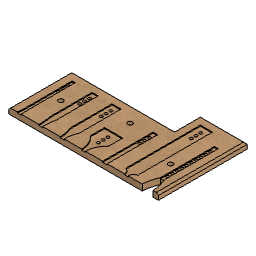
model (Autodesk Fusion 360 design; units mm, degrees)
Autodesk Fusion 360 part; units mm, degrees
(part 1 of 4)
sketch "scan" plane through (0, 0, 0) normal (0, 0, 1) x (1, 0, 0)
  spline S0 degree 3 poles (16.3721, 38.0071) (16.4657, 38.4045) (16.5594, 38.8018) (16.653, 39.1992) knots 0 0 0 0 1 1 1 1
  spline S1 degree 3 poles (24.0485, 109.3811) (21.8648, 109.3248) (19.6635, 109.4946) (17.4974, 109.2121) knots 0 0 0 0 1 1 1 1
  spline S2 degree 3 poles (17.4974, 109.2121) (17.1008, 109.1604) (16.6596, 108.8066) (16.6045, 108.4104) knots 0 0 0 0 1 1 1 1
  spline S3 degree 3 poles (16.6045, 108.4104) (16.3062, 106.2687) (16.4944, 104.0868) (16.4827, 101.9245) knots 0 0 0 0 1 1 1 1
  spline S4 degree 3 poles (16.4827, 101.9245) (16.4424, 94.5014) (16.447, 87.0781) (16.4485, 79.6549) knots 0 0 0 0 1 1 1 1
  spline S5 degree 3 poles (16.4485, 79.6549) (16.4488, 78.5036) (16.4235, 77.3507) (16.4881, 76.2012) knots 0 0 0 0 1 1 1 1
  spline S6 degree 3 poles (16.4881, 76.2012) (16.5002, 75.9869) (16.653, 75.7989) (16.6771, 75.5856) knots 0 0 0 0 1 1 1 1
  spline S7 degree 3 poles (16.6771, 75.5856) (16.7158, 75.2443) (16.6755, 74.8985) (16.6746, 74.555) knots 0 0 0 0 1 1 1 1
  spline S8 degree 3 poles (17.0021, 108.8537) (16.9862, 98.3384) (16.9774, 87.823) (16.9544, 77.3076) knots 0 0 0 0 1 1 1 1
  spline S9 degree 3 poles (16.9544, 77.3076) (16.9536, 76.9758) (16.9724, 76.6416) (16.9307, 76.3123) knots 0 0 0 0 1 1 1 1
  spline S10 degree 3 poles (16.9307, 76.3123) (16.8044, 75.3143) (16.5462, 74.3342) (16.4514, 73.3326) knots 0 0 0 0 1 1 1 1
  spline S11 degree 3 poles (16.4514, 73.3326) (16.3616, 72.3843) (16.3872, 71.4283) (16.378, 70.4757) knots 0 0 0 0 1 1 1 1
  spline S12 degree 3 poles (16.378, 70.4757) (16.3753, 70.1956) (16.3712, 69.9127) (16.4159, 69.6362) knots 0 0 0 0 1 1 1 1
  spline S13 degree 3 poles (16.4159, 69.6362) (16.5418, 68.859) (16.77, 68.1003) (16.8886, 67.322) knots 0 0 0 0 1 1 1 1
  spline S14 degree 3 poles (16.8886, 67.322) (16.9349, 67.018) (16.9083, 66.7072) (16.9093, 66.3996) knots 0 0 0 0 1 1 1 1
  spline S15 degree 3 poles (16.9093, 66.3996) (16.9325, 58.9199) (17.042, 51.4397) (16.9613, 43.9603) knots 0 0 0 0 1 1 1 1
  spline S16 degree 3 poles (16.9613, 43.9603) (16.9556, 43.4252) (16.6548, 42.9203) (16.6502, 42.3851) knots 0 0 0 0 1 1 1 1
  spline S17 degree 3 poles (16.6502, 42.3851) (16.6468, 41.9959) (16.8806, 41.6384) (16.938, 41.2534) knots 0 0 0 0 1 1 1 1
  spline S18 degree 3 poles (16.938, 41.2534) (16.9834, 40.9489) (16.9566, 40.6379) (16.9564, 40.3301) knots 0 0 0 0 1 1 1 1
  spline S19 degree 3 poles (16.9564, 40.3301) (16.9563, 40.2112) (16.9677, 40.0888) (16.9369, 39.9739) knots 0 0 0 0 1 1 1 1
  spline S20 degree 3 poles (16.9369, 39.9739) (16.8656, 39.7083) (16.7476, 39.4575) (16.653, 39.1992) knots 0 0 0 0 1 1 1 1
  spline S21 degree 3 poles (16.674, 74.3159) (16.7683, 73.9813) (16.9278, 73.6585) (16.9568, 73.3121) knots 0 0 0 0 1 1 1 1
  spline S22 degree 3 poles (16.9568, 73.3121) (17.0258, 72.4891) (16.9752, 71.6602) (16.9658, 70.8343) knots 0 0 0 0 1 1 1 1
  spline S23 degree 3 poles (16.9658, 70.8343) (16.9603, 70.3518) (16.993, 69.8634) (16.9124, 69.3876) knots 0 0 0 0 1 1 1 1
  spline S24 degree 3 poles (16.9124, 69.3876) (16.7951, 68.6953) (16.5155, 68.0387) (16.3757, 67.3506) knots 0 0 0 0 1 1 1 1
  spline S25 degree 3 poles (16.3757, 67.3506) (16.3264, 67.1081) (16.3472, 66.8563) (16.3477, 66.6089) knots 0 0 0 0 1 1 1 1
  spline S26 degree 3 poles (16.3477, 66.6089) (16.3626, 59.0903) (16.3279, 51.5712) (16.4218, 44.0531) knots 0 0 0 0 1 1 1 1
  spline S27 degree 3 poles (16.4218, 44.0531) (16.4288, 43.492) (16.6492, 42.9463) (16.6502, 42.3851) knots 0 0 0 0 1 1 1 1
  spline S28 degree 3 poles (16.6502, 42.3851) (16.6512, 41.79) (16.4763, 41.2067) (16.4279, 40.6135) knots 0 0 0 0 1 1 1 1
  spline S29 degree 3 poles (16.4279, 40.6135) (16.41, 40.3942) (16.4182, 40.1712) (16.4517, 39.9536) knots 0 0 0 0 1 1 1 1
  spline S30 degree 3 poles (16.4517, 39.9536) (16.5857, 39.0828) (16.8758, 38.2335) (16.9295, 37.3541) knots 0 0 0 0 1 1 1 1
  spline S31 degree 3 poles (16.9295, 37.3541) (17.0419, 35.5128) (16.9584, 33.6646) (16.9484, 31.8199) knots 0 0 0 0 1 1 1 1
  spline S32 degree 3 poles (16.9484, 31.8199) (16.9468, 31.5315) (16.9648, 31.2361) (16.8948, 30.9563) knots 0 0 0 0 1 1 1 1
  spline S33 degree 3 poles (16.8948, 30.9563) (16.8, 30.5773) (16.605, 30.2306) (16.4602, 29.8678) knots 0 0 0 0 1 1 1 1
  spline S34 degree 3 poles (16.3721, 38.0071) (16.4021, 37.3563) (16.4583, 36.7062) (16.4621, 36.0548) knots 0 0 0 0 1 1 1 1
  spline S35 degree 3 poles (16.4621, 36.0548) (16.4803, 32.9771) (16.3867, 29.8988) (16.4382, 26.8215) knots 0 0 0 0 1 1 1 1
  spline S36 degree 3 poles (16.4382, 26.8215) (16.4474, 26.27) (16.5754, 25.7268) (16.644, 25.1795) knots 0 0 0 0 1 1 1 1
  spline S37 degree 3 poles (16.4626, 31.0645) (16.6175, 30.6597) (16.8137, 30.2684) (16.9274, 29.8501) knots 0 0 0 0 1 1 1 1
  spline S38 degree 3 poles (16.9274, 29.8501) (16.977, 29.6674) (16.9469, 29.4717) (16.9467, 29.2823) knots 0 0 0 0 1 1 1 1
  spline S39 degree 3 poles (16.9467, 29.2823) (16.9452, 28.2612) (16.9973, 27.2375) (16.9222, 26.2193) knots 0 0 0 0 1 1 1 1
  spline S40 degree 3 poles (16.9222, 26.2193) (16.8958, 25.8615) (16.683, 25.5362) (16.644, 25.1795) knots 0 0 0 0 1 1 1 1
  spline S41 degree 3 poles (16.644, 25.1795) (16.5882, 24.6699) (16.6796, 24.1528) (16.64, 23.6417) knots 0 0 0 0 1 1 1 1
  spline S42 degree 3 poles (16.64, 23.6417) (16.6178, 23.3553) (16.4873, 23.0849) (16.4597, 22.799) knots 0 0 0 0 1 1 1 1
  spline S43 degree 3 poles (16.4597, 22.799) (16.3985, 22.1675) (16.3449, 21.5313) (16.3743, 20.8976) knots 0 0 0 0 1 1 1 1
  spline S44 degree 3 poles (16.3743, 20.8976) (16.3993, 20.358) (16.5395, 19.83) (16.6221, 19.2962) knots 0 0 0 0 1 1 1 1
  spline S45 degree 3 poles (15.8229, 0.017) (15.863, 0.507) (15.9277, 0.9956) (15.9433, 1.487) knots 0 0 0 0 1 1 1 1
  spline S46 degree 3 poles (15.9433, 1.487) (16.1106, 6.7611) (16.1154, 12.0409) (16.3715, 17.3114) knots 0 0 0 0 1 1 1 1
  spline S47 degree 3 poles (16.3715, 17.3114) (16.4372, 18.6632) (16.7727, 19.9893) (16.9077, 21.336) knots 0 0 0 0 1 1 1 1
  spline S48 degree 3 poles (16.9077, 21.336) (16.9543, 21.8005) (16.9692, 22.2727) (16.9154, 22.7365) knots 0 0 0 0 1 1 1 1
  spline S49 degree 3 poles (16.9154, 22.7365) (16.879, 23.0498) (16.7318, 23.3399) (16.64, 23.6417) knots 0 0 0 0 1 1 1 1
  spline S50 degree 3 poles (16.33, 0.0256) (16.4989, 5.1912) (16.6867, 10.3561) (16.8367, 15.5223) knots 0 0 0 0 1 1 1 1
  spline S51 degree 3 poles (16.8367, 15.5223) (16.8574, 16.2368) (16.8899, 16.9534) (16.842, 17.6666) knots 0 0 0 0 1 1 1 1
  spline S52 degree 3 poles (16.842, 17.6666) (16.8169, 18.041) (16.6931, 18.4021) (16.6187, 18.7699) knots 0 0 0 0 1 1 1 1
  spline S53 degree 3 poles (23.6843, 24.1713) (23.7833, 24.7166) (23.8823, 25.2618) (23.9813, 25.8071) knots 0 0 0 0 1 1 1 1
  spline S54 degree 3 poles (23.946, 50.5495) (23.8732, 50.1915) (23.7551, 49.8398) (23.7276, 49.4756) knots 0 0 0 0 1 1 1 1
  spline S55 degree 3 poles (23.7276, 49.4756) (23.6586, 48.5602) (23.6607, 47.6406) (23.6575, 46.7227) knots 0 0 0 0 1 1 1 1
  spline S56 degree 3 poles (23.6575, 46.7227) (23.6433, 42.5512) (23.6628, 38.3797) (23.6757, 34.2082) knots 0 0 0 0 1 1 1 1
  spline S57 degree 3 poles (23.6757, 34.2082) (23.6765, 33.9424) (23.637, 33.6698) (23.6985, 33.4112) knots 0 0 0 0 1 1 1 1
  spline S58 degree 3 poles (23.6985, 33.4112) (23.8246, 32.8813) (24.0546, 32.3816) (24.2327, 31.8669) knots 0 0 0 0 1 1 1 1
  spline S59 degree 3 poles (24.1935, 40.1987) (24.0636, 40.2075) (23.9098, 40.1496) (23.8037, 40.2251) knots 0 0 0 0 1 1 1 1
  spline S60 degree 3 poles (23.8037, 40.2251) (23.7167, 40.287) (23.7491, 40.4314) (23.7218, 40.5345) knots 0 0 0 0 1 1 1 1
  spline S61 degree 3 poles (24.2007, 33.6134) (24.0442, 33.0019) (23.8612, 32.3965) (23.7312, 31.7788) knots 0 0 0 0 1 1 1 1
  spline S62 degree 3 poles (23.7312, 31.7788) (23.6859, 31.5639) (23.6512, 31.3404) (23.6764, 31.1222) knots 0 0 0 0 1 1 1 1
  spline S63 degree 3 poles (23.6764, 31.1222) (23.7323, 30.6384) (23.9641, 30.1784) (23.9723, 29.6914) knots 0 0 0 0 1 1 1 1
  spline S64 degree 3 poles (23.9723, 29.6914) (23.9792, 29.2772) (23.7818, 28.8841) (23.7207, 28.4744) knots 0 0 0 0 1 1 1 1
  spline S65 degree 3 poles (23.7207, 28.4744) (23.6825, 28.2188) (23.6372, 27.956) (23.6753, 27.7003) knots 0 0 0 0 1 1 1 1
  spline S66 degree 3 poles (23.6753, 27.7003) (23.7246, 27.3691) (23.8774, 27.0618) (23.9785, 26.7426) knots 0 0 0 0 1 1 1 1
  spline S67 degree 3 poles (23.6843, 24.1713) (23.7003, 23.6899) (23.6664, 23.2041) (23.7324, 22.7269) knots 0 0 0 0 1 1 1 1
  spline S68 degree 3 poles (23.7324, 22.7269) (23.8549, 21.8395) (24.0761, 20.9685) (24.248, 20.0894) knots 0 0 0 0 1 1 1 1
  spline S69 degree 3 poles (23.4385, 100.4157) (23.5823, 100.2547) (23.7636, 100.1207) (23.8699, 99.9329) knots 0 0 0 0 1 1 1 1
  spline S70 degree 3 poles (23.8699, 99.9329) (23.9528, 99.7863) (23.9729, 99.6096) (23.9892, 99.442) knots 0 0 0 0 1 1 1 1
  spline S71 degree 3 poles (23.9892, 99.442) (24.0211, 99.1153) (24.0124, 98.7857) (24.0138, 98.4574) knots 0 0 0 0 1 1 1 1
  spline S72 degree 3 poles (24.0138, 98.4574) (24.0757, 83.7332) (24.1314, 69.009) (24.1791, 54.2847) knots 0 0 0 0 1 1 1 1
  spline S73 degree 3 poles (24.1791, 54.2847) (24.1801, 53.9748) (24.1997, 53.6625) (24.1601, 53.3551) knots 0 0 0 0 1 1 1 1
  spline S74 degree 3 poles (24.1601, 53.3551) (24.1196, 53.041) (23.9645, 52.7466) (23.9404, 52.4308) knots 0 0 0 0 1 1 1 1
  spline S75 degree 3 poles (23.9404, 52.4308) (23.8927, 51.8055) (23.8879, 51.1739) (23.946, 50.5495) knots 0 0 0 0 1 1 1 1
  spline S76 degree 3 poles (23.946, 50.5495) (23.9931, 50.0428) (24.2179, 49.5619) (24.2545, 49.0544) knots 0 0 0 0 1 1 1 1
  spline S77 degree 3 poles (24.2545, 49.0544) (24.2972, 48.4619) (24.1822, 47.8678) (24.1821, 47.2738) knots 0 0 0 0 1 1 1 1
  spline S78 degree 3 poles (24.1821, 47.2738) (24.1818, 41.982) (24.2377, 36.6903) (24.2534, 31.3985) knots 0 0 0 0 1 1 1 1
  spline S79 degree 3 poles (24.2534, 31.3985) (24.2541, 31.1665) (24.269, 30.9318) (24.2313, 30.7028) knots 0 0 0 0 1 1 1 1
  spline S80 degree 3 poles (24.2313, 30.7028) (24.1747, 30.3595) (23.9739, 30.0394) (23.9723, 29.6914) knots 0 0 0 0 1 1 1 1
  spline S81 degree 3 poles (23.9723, 29.6914) (23.9706, 29.3333) (24.1632, 28.9997) (24.2218, 28.6464) knots 0 0 0 0 1 1 1 1
  spline S82 degree 3 poles (24.2218, 28.6464) (24.2517, 28.4657) (24.2597, 28.2787) (24.2364, 28.097) knots 0 0 0 0 1 1 1 1
  spline S83 degree 3 poles (24.2364, 28.097) (24.1782, 27.6411) (24.0318, 27.1991) (23.9785, 26.7426) knots 0 0 0 0 1 1 1 1
  spline S84 degree 3 poles (23.9785, 26.7426) (23.9463, 26.4664) (23.9566, 26.1854) (23.981, 25.9085) knots 0 0 0 0 1 1 1 1
  spline S85 degree 3 poles (23.981, 25.9085) (24.0189, 25.4788) (24.1289, 25.0573) (24.1651, 24.6275) knots 0 0 0 0 1 1 1 1
  spline S86 degree 3 poles (24.1651, 24.6275) (24.2196, 23.9789) (24.3139, 23.3249) (24.2528, 22.6769) knots 0 0 0 0 1 1 1 1
  spline S87 degree 3 poles (24.2528, 22.6769) (24.1883, 21.9925) (23.8437, 21.3522) (23.7917, 20.6667) knots 0 0 0 0 1 1 1 1
  spline S88 degree 3 poles (23.7917, 20.6667) (23.6812, 19.2096) (23.7639, 17.7441) (23.7679, 16.2828) knots 0 0 0 0 1 1 1 1
  spline S89 degree 3 poles (23.7679, 16.2828) (23.7717, 14.862) (23.7838, 13.4412) (23.8152, 12.0208) knots 0 0 0 0 1 1 1 1
  spline S90 degree 3 poles (23.8152, 12.0208) (23.8192, 11.8398) (23.8278, 11.6559) (23.8741, 11.4809) knots 0 0 0 0 1 1 1 1
  spline S91 degree 3 poles (23.8741, 11.4809) (24.013, 10.9556) (24.2038, 10.4454) (24.3687, 9.9276) knots 0 0 0 0 1 1 1 1
  spline S92 degree 3 poles (24.3214, 0.0203) (24.2465, 0.652) (24.1289, 1.2801) (24.0966, 1.9155) knots 0 0 0 0 1 1 1 1
  spline S93 degree 3 poles (24.0966, 1.9155) (23.9822, 4.1649) (23.9401, 6.4174) (23.8815, 8.669) knots 0 0 0 0 1 1 1 1
  spline S94 degree 3 poles (23.8815, 8.669) (23.8707, 9.0818) (23.8364, 9.4981) (23.8885, 9.9077) knots 0 0 0 0 1 1 1 1
  spline S95 degree 3 poles (23.8885, 9.9077) (23.9589, 10.4618) (24.1274, 10.9989) (24.2469, 11.5445) knots 0 0 0 0 1 1 1 1
  spline S96 degree 3 poles (24.4391, 5.607) (24.2812, 5.5747) (24.1233, 5.5424) (23.9655, 5.5101) knots 0 0 0 0 1 1 1 1
  spline S97 degree 3 poles (24.8201, 0.0917) (24.6841, 2.0939) (24.5042, 4.0936) (24.4122, 6.0983) knots 0 0 0 0 1 1 1 1
  spline S98 degree 3 poles (24.4122, 6.0983) (24.3536, 7.3735) (24.4074, 8.6517) (24.3687, 9.9276) knots 0 0 0 0 1 1 1 1
  spline S99 degree 3 poles (24.3687, 9.9276) (24.3523, 10.4678) (24.2522, 11.004) (24.2469, 11.5445) knots 0 0 0 0 1 1 1 1
  spline S100 degree 3 poles (24.2469, 11.5445) (24.2113, 15.2031) (24.2464, 18.8621) (24.2461, 22.5209) knots 0 0 0 0 1 1 1 1
  spline S101 degree 3 poles (23.3873, 100.476) (23.421, 100.0964) (23.4834, 99.7184) (23.4883, 99.3374) knots 0 0 0 0 1 1 1 1
  spline S102 degree 3 poles (23.4883, 99.3374) (23.5251, 96.5129) (23.4778, 93.6877) (23.5126, 90.8631) knots 0 0 0 0 1 1 1 1
  spline S103 degree 3 poles (23.5126, 90.8631) (23.5222, 90.0839) (23.6184, 89.3072) (23.6216, 88.5279) knots 0 0 0 0 1 1 1 1
  spline S104 degree 3 poles (23.6216, 88.5279) (23.623, 88.202) (23.5263, 87.8808) (23.5264, 87.5549) knots 0 0 0 0 1 1 1 1
  spline S105 degree 3 poles (23.5264, 87.5549) (23.5273, 85.3803) (23.5604, 83.2055) (23.6246, 81.0319) knots 0 0 0 0 1 1 1 1
  spline S106 degree 3 poles (23.6246, 81.0319) (23.6322, 80.7737) (23.6228, 80.4951) (23.7418, 80.2659) knots 0 0 0 0 1 1 1 1
  spline S107 degree 3 poles (23.7418, 80.2659) (23.7992, 80.1554) (23.9747, 80.1777) (24.0911, 80.1336) knots 0 0 0 0 1 1 1 1
  spline S108 degree 3 poles (24.0789, 79.6378) (23.9819, 79.6107) (23.8527, 79.6337) (23.7881, 79.5565) knots 0 0 0 0 1 1 1 1
  spline S109 degree 3 poles (23.7881, 79.5565) (23.7115, 79.4651) (23.7209, 79.325) (23.7168, 79.2058) knots 0 0 0 0 1 1 1 1
  spline S110 degree 3 poles (23.7168, 79.2058) (23.67, 77.8254) (23.6398, 76.4443) (23.6357, 75.0631) knots 0 0 0 0 1 1 1 1
  spline S111 degree 3 poles (23.6357, 75.0631) (23.6143, 67.9218) (23.5442, 60.7797) (23.6404, 53.6389) knots 0 0 0 0 1 1 1 1
  spline S112 degree 3 poles (23.6404, 53.6389) (23.646, 53.224) (23.8404, 52.8335) (23.9404, 52.4308) knots 0 0 0 0 1 1 1 1
  spline S113 degree 3 poles (38.0415, 3.3563) (38.0887, 2.9587) (38.136, 2.5612) (38.1832, 2.1637) knots 0 0 0 0 1 1 1 1
  spline S114 degree 3 poles (37.1611, 15.8815) (37.0742, 15.8569) (36.9605, 15.8752) (36.9005, 15.8078) knots 0 0 0 0 1 1 1 1
  spline S115 degree 3 poles (36.9005, 15.8078) (36.799, 15.6939) (36.7805, 15.5273) (36.7206, 15.387) knots 0 0 0 0 1 1 1 1
  spline S116 degree 3 poles (35.4592, 92.8027) (35.5064, 92.9064) (35.5536, 93.0101) (35.6007, 93.1139) knots 0 0 0 0 1 1 1 1
  spline S117 degree 3 poles (48.9333, 95.3582) (49.0217, 94.9561) (49.1322, 94.5582) (49.1985, 94.1519) knots 0 0 0 0 1 1 1 1
  spline S118 degree 3 poles (49.1985, 94.1519) (49.2367, 93.9176) (49.2439, 93.6787) (49.246, 93.4413) knots 0 0 0 0 1 1 1 1
  spline S119 degree 3 poles (49.246, 93.4413) (49.2753, 89.9902) (49.2842, 86.539) (49.2926, 83.0877) knots 0 0 0 0 1 1 1 1
  spline S120 degree 3 poles (49.2926, 83.0877) (49.2954, 81.9165) (49.3382, 80.7437) (49.2797, 79.5739) knots 0 0 0 0 1 1 1 1
  spline S121 degree 3 poles (49.2797, 79.5739) (49.2036, 78.0516) (48.9932, 76.5386) (48.889, 75.0179) knots 0 0 0 0 1 1 1 1
  spline S122 degree 3 poles (48.889, 75.0179) (48.8593, 74.5836) (48.876, 74.1473) (48.878, 73.712) knots 0 0 0 0 1 1 1 1
  spline S123 degree 3 poles (48.878, 73.712) (48.9551, 57.4318) (49.1081, 41.1519) (49.1263, 24.8715) knots 0 0 0 0 1 1 1 1
  spline S124 degree 3 poles (49.1263, 24.8715) (49.1274, 23.8581) (49.0563, 22.8434) (48.9359, 21.8372) knots 0 0 0 0 1 1 1 1
  spline S125 degree 3 poles (48.9359, 21.8372) (48.6206, 19.2034) (48.0478, 16.6008) (47.8198, 13.958) knots 0 0 0 0 1 1 1 1
  spline S126 degree 3 poles (47.8198, 13.958) (47.7658, 13.3326) (48.1088, 12.7227) (48.0952, 12.0951) knots 0 0 0 0 1 1 1 1
  spline S127 degree 3 poles (48.0952, 12.0951) (48.0605, 10.4936) (47.8155, 8.9035) (47.6756, 7.3076) knots 0 0 0 0 1 1 1 1
  spline S128 degree 3 poles (48.6864, 16.6735) (48.5207, 16.7022) (48.3549, 16.731) (48.1891, 16.7597) knots 0 0 0 0 1 1 1 1
  spline S129 degree 3 poles (49.1012, 76.8549) (49.1913, 76.2486) (49.3076, 75.6455) (49.3715, 75.0358) knots 0 0 0 0 1 1 1 1
  spline S130 degree 3 poles (49.3715, 75.0358) (49.4035, 74.7298) (49.3869, 74.4206) (49.3884, 74.1129) knots 0 0 0 0 1 1 1 1
  spline S131 degree 3 poles (49.3884, 74.1129) (49.4723, 57.1953) (49.6539, 40.2779) (49.6278, 23.3602) knots 0 0 0 0 1 1 1 1
  spline S132 degree 3 poles (49.6278, 23.3602) (49.6264, 22.448) (49.378, 21.552) (49.3059, 20.6426) knots 0 0 0 0 1 1 1 1
  spline S133 degree 3 poles (49.3059, 20.6426) (49.2968, 20.5279) (49.4053, 20.4201) (49.3856, 20.3068) knots 0 0 0 0 1 1 1 1
  spline S134 degree 3 poles (49.3856, 20.3068) (49.3322, 19.9995) (49.1435, 19.7259) (49.0931, 19.4181) knots 0 0 0 0 1 1 1 1
  spline S135 degree 3 poles (49.0931, 19.4181) (48.7846, 17.5331) (48.6884, 15.6139) (48.3112, 13.7415) knots 0 0 0 0 1 1 1 1
  spline S136 degree 3 poles (48.3112, 13.7415) (48.1679, 13.0303) (47.6736, 12.4196) (47.5394, 11.7067) knots 0 0 0 0 1 1 1 1
  spline S137 degree 3 poles (47.5394, 11.7067) (47.3273, 10.5797) (47.2469, 9.4223) (47.2824, 8.2761) knots 0 0 0 0 1 1 1 1
  spline S138 degree 3 poles (47.2824, 8.2761) (47.2932, 7.9279) (47.644, 7.6546) (47.6756, 7.3076) knots 0 0 0 0 1 1 1 1
  spline S139 degree 3 poles (47.6756, 7.3076) (47.7327, 6.6813) (47.5866, 6.053) (47.5421, 5.4256) knots 0 0 0 0 1 1 1 1
  spline S140 degree 3 poles (46.8789, -0.0661) (46.9136, 1.4443) (46.9101, 2.9561) (46.9831, 4.4652) knots 0 0 0 0 1 1 1 1
  spline S141 degree 3 poles (46.9831, 4.4652) (47.0447, 5.738) (47.1827, 7.0058) (47.2824, 8.2761) knots 0 0 0 0 1 1 1 1
  spline S142 degree 3 poles (47.3881, 0.0661) (47.4395, 1.8526) (47.6025, 3.6394) (47.5421, 5.4256) knots 0 0 0 0 1 1 1 1
  spline S143 degree 3 poles (47.5421, 5.4256) (47.5265, 5.887) (47.2887, 6.3134) (47.162, 6.7573) knots 0 0 0 0 1 1 1 1
  spline S144 degree 3 poles (49.6954, 18.6702) (49.4724, 18.6205) (49.2493, 18.5708) (49.0262, 18.521) knots 0 0 0 0 1 1 1 1
  spline S145 degree 3 poles (42.2923, 109.9049) (41.941, 109.9745) (41.5954, 110.0838) (41.2386, 110.1137) knots 0 0 0 0 1 1 1 1
  spline S146 degree 3 poles (41.2386, 110.1137) (40.735, 110.1558) (40.2266, 110.157) (39.7226, 110.1201) knots 0 0 0 0 1 1 1 1
  spline S147 degree 3 poles (39.7226, 110.1201) (39.3754, 110.0947) (39.0422, 109.9656) (38.6963, 109.9275) knots 0 0 0 0 1 1 1 1
  spline S148 degree 3 poles (38.6963, 109.9275) (38.4842, 109.9041) (38.2678, 109.9642) (38.0563, 109.9364) knots 0 0 0 0 1 1 1 1
  spline S149 degree 3 poles (38.0563, 109.9364) (37.756, 109.8969) (37.4728, 109.7626) (37.1719, 109.727) knots 0 0 0 0 1 1 1 1
  spline S150 degree 3 poles (37.1719, 109.727) (36.7902, 109.6818) (36.3971, 109.6246) (36.0192, 109.6952) knots 0 0 0 0 1 1 1 1
  spline S151 degree 3 poles (36.0192, 109.6952) (35.8914, 109.719) (35.8299, 109.878) (35.7638, 109.99) knots 0 0 0 0 1 1 1 1
  spline S152 degree 3 poles (35.7638, 109.99) (35.7262, 110.0537) (35.7326, 110.1347) (35.717, 110.207) knots 0 0 0 0 1 1 1 1
  spline S153 degree 3 poles (38.0563, 109.9364) (37.6106, 110.077) (37.1859, 110.3328) (36.7192, 110.358) knots 0 0 0 0 1 1 1 1
  spline S154 degree 3 poles (36.7192, 110.358) (36.209, 110.3857) (35.7011, 110.2311) (35.2098, 110.0906) knots 0 0 0 0 1 1 1 1
  spline S155 degree 3 poles (35.2098, 110.0906) (35.1184, 110.0644) (35.0262, 109.9685) (35.025, 109.8734) knots 0 0 0 0 1 1 1 1
  spline S156 degree 3 poles (35.025, 109.8734) (34.9724, 105.9862) (35.0226, 102.0982) (35.0492, 98.2108) knots 0 0 0 0 1 1 1 1
  spline S157 degree 3 poles (35.0492, 98.2108) (35.0507, 98.001) (35.0445, 97.7838) (35.109, 97.5842) knots 0 0 0 0 1 1 1 1
  spline S158 degree 3 poles (35.109, 97.5842) (35.2282, 97.2156) (35.4318, 96.88) (35.5932, 96.5279) knots 0 0 0 0 1 1 1 1
  spline S159 degree 3 poles (35.2427, 92.7971) (35.1944, 93.0635) (35.1091, 93.3258) (35.0977, 93.5964) knots 0 0 0 0 1 1 1 1
  spline S160 degree 3 poles (35.0977, 93.5964) (35.0595, 94.4984) (34.9988, 95.4071) (35.0942, 96.305) knots 0 0 0 0 1 1 1 1
  spline S161 degree 3 poles (35.0942, 96.305) (35.1484, 96.8153) (35.3926, 97.287) (35.5418, 97.778) knots 0 0 0 0 1 1 1 1
  spline S162 degree 3 poles (35.0977, 93.5964) (35.1135, 89.6975) (35.05, 85.7975) (35.1453, 81.8998) knots 0 0 0 0 1 1 1 1
  spline S163 degree 3 poles (35.1453, 81.8998) (35.157, 81.4206) (35.3272, 80.9584) (35.4181, 80.4877) knots 0 0 0 0 1 1 1 1
  spline S164 degree 3 poles (35.6281, 83.4219) (35.4749, 83.4274) (35.3218, 83.4329) (35.1686, 83.4383) knots 0 0 0 0 1 1 1 1
  spline S165 degree 3 poles (35.4269, 79.0966) (35.342, 78.8264) (35.2228, 78.5646) (35.1722, 78.286) knots 0 0 0 0 1 1 1 1
  spline S166 degree 3 poles (35.1722, 78.286) (35.1307, 78.0573) (35.1526, 77.8215) (35.1533, 77.5891) knots 0 0 0 0 1 1 1 1
  spline S167 degree 3 poles (35.1533, 77.5891) (35.1541, 77.357) (35.139, 77.1222) (35.1766, 76.8932) knots 0 0 0 0 1 1 1 1
  spline S168 degree 3 poles (35.1766, 76.8932) (35.2374, 76.523) (35.3569, 76.1649) (35.447, 75.8008) knots 0 0 0 0 1 1 1 1
  spline S169 degree 3 poles (35.4556, 74.3617) (35.3609, 74.1057) (35.1745, 73.8667) (35.1717, 73.5938) knots 0 0 0 0 1 1 1 1
  spline S170 degree 3 poles (35.1717, 73.5938) (35.1231, 68.7942) (35.2458, 63.9943) (35.3021, 59.1948) knots 0 0 0 0 1 1 1 1
  spline S171 degree 3 poles (35.3021, 59.1948) (35.3048, 58.9612) (35.306, 58.7252) (35.3487, 58.4955) knots 0 0 0 0 1 1 1 1
  spline S172 degree 3 poles (35.3487, 58.4955) (35.3925, 58.2594) (35.5635, 58.0468) (35.5598, 57.8066) knots 0 0 0 0 1 1 1 1
  spline S173 degree 3 poles (35.5598, 57.8066) (35.5561, 57.5669) (35.3723, 57.3614) (35.3276, 57.1259) knots 0 0 0 0 1 1 1 1
  spline S174 degree 3 poles (35.3276, 57.1259) (35.2797, 56.8734) (35.2881, 56.6132) (35.2845, 56.3563) knots 0 0 0 0 1 1 1 1
  spline S175 degree 3 poles (35.2845, 56.3563) (35.2815, 56.1421) (35.2756, 55.9258) (35.308, 55.7141) knots 0 0 0 0 1 1 1 1
  spline S176 degree 3 poles (35.308, 55.7141) (35.3756, 55.2727) (35.4918, 54.8401) (35.5837, 54.4031) knots 0 0 0 0 1 1 1 1
  spline S177 degree 3 poles (35.7638, 109.99) (35.7072, 109.7297) (35.6086, 109.475) (35.594, 109.209) knots 0 0 0 0 1 1 1 1
  spline S178 degree 3 poles (35.594, 109.209) (35.531, 108.066) (35.529, 106.9201) (35.5316, 105.7754) knots 0 0 0 0 1 1 1 1
  spline S179 degree 3 poles (35.5316, 105.7754) (35.5497, 97.8944) (35.6914, 90.0136) (35.6561, 82.1326) knots 0 0 0 0 1 1 1 1
  spline S180 degree 3 poles (35.6561, 82.1326) (35.6536, 81.5786) (35.4598, 81.0402) (35.4181, 80.4877) knots 0 0 0 0 1 1 1 1
  spline S181 degree 3 poles (35.4181, 80.4877) (35.3832, 80.0253) (35.3799, 79.5579) (35.4269, 79.0966) knots 0 0 0 0 1 1 1 1
  spline S182 degree 3 poles (35.4269, 79.0966) (35.4618, 78.7532) (35.6275, 78.4316) (35.6622, 78.0882) knots 0 0 0 0 1 1 1 1
  spline S183 degree 3 poles (35.6622, 78.0882) (35.7028, 77.6879) (35.6889, 77.2818) (35.6512, 76.8812) knots 0 0 0 0 1 1 1 1
  spline S184 degree 3 poles (35.6512, 76.8812) (35.6168, 76.5163) (35.4753, 76.1662) (35.447, 75.8008) knots 0 0 0 0 1 1 1 1
  spline S185 degree 3 poles (35.447, 75.8008) (35.4098, 75.3225) (35.4077, 74.839) (35.4556, 74.3617) knots 0 0 0 0 1 1 1 1
  spline S186 degree 3 poles (35.4556, 74.3617) (35.4794, 74.1235) (35.6149, 73.9084) (35.6603, 73.6734) knots 0 0 0 0 1 1 1 1
  spline S187 degree 3 poles (35.6603, 73.6734) (35.7026, 73.4544) (35.7128, 73.2296) (35.7175, 73.0066) knots 0 0 0 0 1 1 1 1
  spline S188 degree 3 poles (35.7175, 73.0066) (35.7447, 71.7063) (35.7508, 70.4057) (35.7558, 69.1052) knots 0 0 0 0 1 1 1 1
  spline S189 degree 3 poles (35.7558, 69.1052) (35.7685, 65.8369) (35.8272, 62.568) (35.7705, 59.3001) knots 0 0 0 0 1 1 1 1
  spline S190 degree 3 poles (35.7705, 59.3001) (35.7618, 58.7975) (35.5575, 58.3094) (35.5598, 57.8066) knots 0 0 0 0 1 1 1 1
  spline S191 degree 3 poles (35.5598, 57.8066) (35.561, 57.5312) (35.7434, 57.2834) (35.7808, 57.0105) knots 0 0 0 0 1 1 1 1
  spline S192 degree 3 poles (35.7808, 57.0105) (35.8253, 56.685) (35.8285, 56.3528) (35.8037, 56.0252) knots 0 0 0 0 1 1 1 1
  spline S193 degree 3 poles (35.8037, 56.0252) (35.7626, 55.4811) (35.6334, 54.9465) (35.5837, 54.4031) knots 0 0 0 0 1 1 1 1
  spline S194 degree 3 poles (35.5837, 54.4031) (35.4904, 53.384) (35.3828, 52.3634) (35.3747, 51.34) knots 0 0 0 0 1 1 1 1
  spline S195 degree 3 poles (35.3747, 51.34) (35.3289, 45.5149) (35.3132, 39.6885) (35.422, 33.8643) knots 0 0 0 0 1 1 1 1
  spline S196 degree 3 poles (35.422, 33.8643) (35.4311, 33.3764) (35.7144, 32.9205) (35.7278, 32.4327) knots 0 0 0 0 1 1 1 1
  spline S197 degree 3 poles (35.7278, 32.4327) (35.7399, 31.9906) (35.5077, 31.5682) (35.4973, 31.1261) knots 0 0 0 0 1 1 1 1
  spline S198 degree 3 poles (35.4973, 31.1261) (35.4439, 28.856) (35.4978, 26.5844) (35.5369, 24.3141) knots 0 0 0 0 1 1 1 1
  spline S199 degree 3 poles (35.5369, 24.3141) (35.548, 23.6698) (35.5631, 23.023) (35.6478, 22.3843) knots 0 0 0 0 1 1 1 1
  spline S200 degree 3 poles (35.6478, 22.3843) (35.958, 20.0451) (36.3979, 17.7245) (36.7206, 15.387) knots 0 0 0 0 1 1 1 1
  spline S201 degree 3 poles (36.7206, 15.387) (36.9317, 13.8579) (37.1244, 12.325) (37.249, 10.7865) knots 0 0 0 0 1 1 1 1
  spline S202 degree 3 poles (37.249, 10.7865) (37.4789, 7.9483) (37.6358, 5.1044) (37.784, 2.2608) knots 0 0 0 0 1 1 1 1
  spline S203 degree 3 poles (37.784, 2.2608) (37.818, 1.6078) (37.7917, 0.9531) (37.7956, 0.2992) knots 0 0 0 0 1 1 1 1
  spline S204 degree 3 poles (38.154, 0.1104) (38.1812, 1.4051) (38.2819, 2.7004) (38.2355, 3.9946) knots 0 0 0 0 1 1 1 1
  spline S205 degree 3 poles (38.2355, 3.9946) (38.1462, 6.4866) (38.0227, 8.9812) (37.7471, 11.4596) knots 0 0 0 0 1 1 1 1
  spline S206 degree 3 poles (37.7471, 11.4596) (37.3294, 15.2151) (36.6124, 18.9323) (36.1568, 22.6833) knots 0 0 0 0 1 1 1 1
  spline S207 degree 3 poles (36.1568, 22.6833) (36.0405, 23.6405) (36.0504, 24.6093) (36.0327, 25.5734) knots 0 0 0 0 1 1 1 1
  spline S208 degree 3 poles (36.0327, 25.5734) (35.9975, 27.4915) (36.083, 29.412) (35.9978, 31.3285) knots 0 0 0 0 1 1 1 1
  spline S209 degree 3 poles (35.9978, 31.3285) (35.981, 31.7071) (35.7378, 32.0539) (35.7278, 32.4327) knots 0 0 0 0 1 1 1 1
  spline S210 degree 3 poles (35.7278, 32.4327) (35.7177, 32.8172) (35.9327, 33.1825) (35.9389, 33.567) knots 0 0 0 0 1 1 1 1
  spline S211 degree 3 poles (35.9389, 33.567) (35.9914, 36.8137) (36.0508, 40.0646) (35.9036, 43.3084) knots 0 0 0 0 1 1 1 1
  spline S212 degree 3 poles (35.9036, 43.3084) (35.8779, 43.8744) (35.5832, 44.3953) (35.423, 44.9387) knots 0 0 0 0 1 1 1 1
  spline S213 degree 3 poles (35.5893, 53.6509) (35.684, 53.047) (35.8548, 52.4502) (35.8733, 51.8392) knots 0 0 0 0 1 1 1 1
  spline S214 degree 3 poles (35.8733, 51.8392) (35.9588, 49.0253) (35.8916, 46.2089) (35.9007, 43.3937) knots 0 0 0 0 1 1 1 1
  spline S215 degree 3 poles (38.6963, 109.9275) (38.9001, 109.9077) (39.1093, 109.9184) (39.3079, 109.8682) knots 0 0 0 0 1 1 1 1
  spline S216 degree 3 poles (39.3079, 109.8682) (39.4601, 109.8298) (39.5773, 109.6843) (39.7331, 109.6657) knots 0 0 0 0 1 1 1 1
  spline S217 degree 3 poles (39.7331, 109.6657) (40.1884, 109.6116) (40.6519, 109.6115) (41.1084, 109.6542) knots 0 0 0 0 1 1 1 1
  spline S218 degree 3 poles (41.1084, 109.6542) (41.51, 109.6917) (41.8899, 109.8761) (42.2923, 109.9049) knots 0 0 0 0 1 1 1 1
  spline S219 degree 3 poles (42.2923, 109.9049) (43.0108, 109.9565) (43.7342, 109.853) (44.4534, 109.8942) knots 0 0 0 0 1 1 1 1
  spline S220 degree 3 poles (44.4534, 109.8942) (44.9381, 109.9219) (45.4091, 110.079) (45.8935, 110.1111) knots 0 0 0 0 1 1 1 1
  spline S221 degree 3 poles (45.8935, 110.1111) (46.505, 110.1517) (47.1193, 110.119) (47.7321, 110.1116) knots 0 0 0 0 1 1 1 1
  spline S222 degree 3 poles (47.7321, 110.1116) (47.8757, 110.1099) (48.0263, 110.1308) (48.162, 110.084) knots 0 0 0 0 1 1 1 1
  spline S223 degree 3 poles (48.162, 110.084) (48.404, 110.0005) (48.7176, 109.9518) (48.8426, 109.7285) knots 0 0 0 0 1 1 1 1
  spline S224 degree 3 poles (48.8426, 109.7285) (49.0295, 109.3945) (48.985, 108.9734) (48.9979, 108.5909) knots 0 0 0 0 1 1 1 1
  spline S225 degree 3 poles (48.9979, 108.5909) (49.0841, 106.0392) (49.1086, 103.4858) (49.1394, 100.933) knots 0 0 0 0 1 1 1 1
  spline S226 degree 3 poles (49.1394, 100.933) (49.1533, 99.783) (49.1842, 98.6317) (49.1323, 97.4829) knots 0 0 0 0 1 1 1 1
  spline S227 degree 3 poles (49.1323, 97.4829) (49.1127, 97.0483) (48.9945, 96.6239) (48.9256, 96.1944) knots 0 0 0 0 1 1 1 1
  spline S228 degree 3 poles (44.4534, 109.8942) (44.7519, 109.8855) (45.0549, 109.9206) (45.3489, 109.8682) knots 0 0 0 0 1 1 1 1
  spline S229 degree 3 poles (45.3489, 109.8682) (45.5435, 109.8336) (45.6983, 109.6555) (45.8952, 109.6373) knots 0 0 0 0 1 1 1 1
  spline S230 degree 3 poles (45.8952, 109.6373) (46.742, 109.5588) (47.5957, 109.5999) (48.446, 109.5813) knots 0 0 0 0 1 1 1 1
  spline S231 degree 3 poles (48.436, 109.9663) (48.4626, 109.1066) (48.4025, 108.2398) (48.5157, 107.3872) knots 0 0 0 0 1 1 1 1
  spline S232 degree 3 poles (48.5157, 107.3872) (48.6184, 106.6135) (48.8918, 105.8723) (49.0798, 105.1148) knots 0 0 0 0 1 1 1 1
  spline S233 degree 3 poles (48.9986, 107.3847) (48.8399, 106.8367) (48.5432, 106.3108) (48.5226, 105.7407) knots 0 0 0 0 1 1 1 1
  spline S234 degree 3 poles (48.5226, 105.7407) (48.4265, 103.0845) (48.5387, 100.4235) (48.6507, 97.768) knots 0 0 0 0 1 1 1 1
  spline S235 degree 3 poles (48.6507, 97.768) (48.6732, 97.236) (48.8635, 96.7233) (48.9256, 96.1944) knots 0 0 0 0 1 1 1 1
  spline S236 degree 3 poles (48.9256, 96.1944) (48.958, 95.9176) (48.9535, 95.6363) (48.9333, 95.3582) knots 0 0 0 0 1 1 1 1
  spline S237 degree 3 poles (48.9333, 95.3582) (48.8843, 94.6817) (48.7242, 94.013) (48.7182, 93.3348) knots 0 0 0 0 1 1 1 1
  spline S238 degree 3 poles (48.7182, 93.3348) (48.6792, 88.9163) (48.7621, 84.4975) (48.7984, 80.079) knots 0 0 0 0 1 1 1 1
  spline S239 degree 3 poles (48.7984, 80.079) (48.8009, 79.7786) (48.7962, 79.4766) (48.8344, 79.1786) knots 0 0 0 0 1 1 1 1
  spline S240 degree 3 poles (48.8344, 79.1786) (48.8949, 78.7064) (49.0074, 78.2422) (49.094, 77.774) knots 0 0 0 0 1 1 1 1
  spline S241 degree 3 poles (49.2086, 91.6123) (49.1552, 91.7) (49.1391, 91.8275) (49.0482, 91.8754) knots 0 0 0 0 1 1 1 1
  spline S242 degree 3 poles (49.0482, 91.8754) (48.9639, 91.9199) (48.8583, 91.8566) (48.7634, 91.8472) knots 0 0 0 0 1 1 1 1
  spline S243 degree 3 poles (49.4712, 58.1439) (49.3033, 58.1202) (49.1354, 58.0966) (48.9676, 58.073) knots 0 0 0 0 1 1 1 1
  spline S244 degree 3 poles (49.4887, 50.5389) (49.3261, 50.582) (49.1636, 50.6251) (49.0011, 50.6681) knots 0 0 0 0 1 1 1 1
  spline S245 degree 3 poles (49.5363, 37.9815) (49.3818, 37.9725) (49.2272, 37.9635) (49.0727, 37.9545) knots 0 0 0 0 1 1 1 1
  spline S246 degree 3 poles (49.5842, 32.8051) (49.4801, 32.7797) (49.3361, 32.8148) (49.2721, 32.729) knots 0 0 0 0 1 1 1 1
  spline S247 degree 3 poles (49.2721, 32.729) (49.1505, 32.5659) (49.1524, 32.3401) (49.0925, 32.1456) knots 0 0 0 0 1 1 1 1
  spline S248 degree 3 poles (49.1858, 19.6824) (49.642, 19.82) (50.1037, 19.9407) (50.5545, 20.0952) knots 0 0 0 0 1 1 1 1
  spline S249 degree 3 poles (50.5545, 20.0952) (50.6132, 20.1153) (50.6738, 20.1504) (50.7061, 20.2034) knots 0 0 0 0 1 1 1 1
  spline S250 degree 3 poles (50.7061, 20.2034) (50.7439, 20.2654) (50.7766, 20.3489) (50.7505, 20.4166) knots 0 0 0 0 1 1 1 1
  spline S251 degree 3 poles (50.7505, 20.4166) (50.7261, 20.4799) (50.6484, 20.5235) (50.5808, 20.529) knots 0 0 0 0 1 1 1 1
  spline S252 degree 3 poles (50.5808, 20.529) (50.165, 20.5627) (49.7464, 20.531) (49.3292, 20.532) knots 0 0 0 0 1 1 1 1
  spline S253 degree 3 poles (37.8384, 151.6265) (37.6193, 151.7633) (37.4002, 151.9002) (37.1811, 152.0371) knots 0 0 0 0 1 1 1 1
  spline S254 degree 3 poles (75.5294, 110.1328) (75.2113, 110.1491) (74.8931, 110.1655) (74.5749, 110.1818) knots 0 0 0 0 1 1 1 1
  spline S255 degree 3 poles (62.4148, 110.2651) (62.1158, 110.2785) (61.8168, 110.2919) (61.5178, 110.3054) knots 0 0 0 0 1 1 1 1
  spline S256 degree 3 poles (64.8858, 3.1426) (64.895, 3.9918) (64.9042, 4.841) (64.9134, 5.6902) knots 0 0 0 0 1 1 1 1
  spline S257 degree 3 poles (64.6058, 5.1109) (64.7083, 5.304) (64.8109, 5.4971) (64.9134, 5.6902) knots 0 0 0 0 1 1 1 1
  spline S258 degree 3 poles (64.7471, 4.2202) (64.8026, 4.7102) (64.858, 5.2002) (64.9134, 5.6902) knots 0 0 0 0 1 1 1 1
  spline S259 degree 3 poles (65.2058, -0.0661) (65.162, 0.6745) (65.0386, 1.4147) (65.0744, 2.1558) knots 0 0 0 0 1 1 1 1
  spline S260 degree 3 poles (65.0744, 2.1558) (65.0929, 2.539) (65.2695, 2.8977) (65.3671, 3.2687) knots 0 0 0 0 1 1 1 1
  spline S261 degree 3 poles (65.5884, 0.2094) (65.5146, 1.2292) (65.5006, 2.255) (65.3671, 3.2687) knots 0 0 0 0 1 1 1 1
  spline S262 degree 3 poles (65.3671, 3.2687) (65.2455, 4.1919) (64.9772, 5.0904) (64.8244, 6.009) knots 0 0 0 0 1 1 1 1
  spline S263 degree 3 poles (64.8244, 6.009) (64.701, 6.7503) (64.6876, 7.5086) (64.5391, 8.2452) knots 0 0 0 0 1 1 1 1
  spline S264 degree 3 poles (64.5391, 8.2452) (64.4346, 8.7638) (64.2251, 9.2556) (64.0681, 9.7608) knots 0 0 0 0 1 1 1 1
  spline S265 degree 3 poles (62.4148, 110.2651) (62.5696, 110.1899) (62.7108, 110.0748) (62.8792, 110.0394) knots 0 0 0 0 1 1 1 1
  spline S266 degree 3 poles (62.8792, 110.0394) (63.1143, 109.9901) (63.3593, 110.017) (63.5996, 110.0162) knots 0 0 0 0 1 1 1 1
  spline S267 degree 3 poles (63.5996, 110.0162) (63.8619, 110.0153) (64.1284, 109.9867) (64.3864, 110.0345) knots 0 0 0 0 1 1 1 1
  spline S268 degree 3 poles (64.3864, 110.0345) (64.5993, 110.0738) (64.7891, 110.1938) (64.9904, 110.2735) knots 0 0 0 0 1 1 1 1
  spline S269 degree 3 poles (77.1922, 110.3761) (77.1922, 110.2208) (77.1922, 110.0655) (77.1922, 109.9102) knots 0 0 0 0 1 1 1 1
  spline S270 degree 3 poles (75.5294, 110.1328) (75.6579, 110.0609) (75.7683, 109.9304) (75.915, 109.9172) knots 0 0 0 0 1 1 1 1
  spline S271 degree 3 poles (75.915, 109.9172) (76.8069, 109.8371) (77.7053, 109.8479) (78.6007, 109.857) knots 0 0 0 0 1 1 1 1
  spline S272 degree 3 poles (78.6007, 109.857) (78.8379, 109.8595) (79.069, 109.9639) (79.3059, 109.9518) knots 0 0 0 0 1 1 1 1
  spline S273 degree 3 poles (79.3059, 109.9518) (79.6461, 109.9345) (80.0256, 109.9553) (80.3113, 109.7698) knots 0 0 0 0 1 1 1 1
  spline S274 degree 3 poles (80.3113, 109.7698) (80.5216, 109.6333) (80.5261, 109.3166) (80.6335, 109.09) knots 0 0 0 0 1 1 1 1
  spline S275 degree 3 poles (58.688, 111.0959) (59.054, 110.9243) (59.3976, 110.6928) (59.7861, 110.581) knots 0 0 0 0 1 1 1 1
  spline S276 degree 3 poles (59.7861, 110.581) (60.3208, 110.4272) (60.8761, 110.3129) (61.4325, 110.3062) knots 0 0 0 0 1 1 1 1
  spline S277 degree 3 poles (61.4325, 110.3062) (62.1471, 110.2975) (62.8513, 110.4861) (63.5643, 110.5351) knots 0 0 0 0 1 1 1 1
  spline S278 degree 3 poles (63.5643, 110.5351) (63.8388, 110.554) (64.1187, 110.559) (64.3894, 110.5094) knots 0 0 0 0 1 1 1 1
  spline S279 degree 3 poles (64.3894, 110.5094) (64.6011, 110.4706) (64.7753, 110.2804) (64.9904, 110.2735) knots 0 0 0 0 1 1 1 1
  spline S280 degree 3 poles (64.9904, 110.2735) (68.1837, 110.1708) (71.3801, 110.1465) (74.5749, 110.1818) knots 0 0 0 0 1 1 1 1
  spline S281 degree 3 poles (74.5749, 110.1818) (75.2677, 110.1894) (75.9504, 110.3572) (76.6418, 110.402) knots 0 0 0 0 1 1 1 1
  spline S282 degree 3 poles (76.6418, 110.402) (77.3324, 110.4469) (78.0264, 110.4095) (78.7172, 110.4506) knots 0 0 0 0 1 1 1 1
  spline S283 degree 3 poles (78.7172, 110.4506) (78.8024, 110.4557) (78.8978, 110.4785) (78.9572, 110.5398) knots 0 0 0 0 1 1 1 1
  spline S284 degree 3 poles (78.9572, 110.5398) (79.0216, 110.6062) (78.9918, 110.7322) (79.0554, 110.7994) knots 0 0 0 0 1 1 1 1
  spline S285 degree 3 poles (79.0554, 110.7994) (79.1105, 110.8576) (79.2073, 110.913) (79.2812, 110.8819) knots 0 0 0 0 1 1 1 1
  spline S286 degree 3 poles (79.2812, 110.8819) (79.4049, 110.8297) (79.5044, 110.7116) (79.5565, 110.5879) knots 0 0 0 0 1 1 1 1
  spline S287 degree 3 poles (79.5565, 110.5879) (79.6452, 110.3775) (79.6443, 110.1397) (79.6881, 109.9157) knots 0 0 0 0 1 1 1 1
  spline S288 degree 3 poles (59.0386, 110.4305) (59.1421, 110.383) (59.2456, 110.3355) (59.3492, 110.2881) knots 0 0 0 0 1 1 1 1
  spline S289 degree 3 poles (59.9293, 77.1959) (59.8952, 86.1006) (59.895, 95.0055) (59.8271, 103.9101) knots 0 0 0 0 1 1 1 1
  spline S290 degree 3 poles (59.8271, 103.9101) (59.8202, 104.8238) (59.7882, 105.7386) (59.7048, 106.6485) knots 0 0 0 0 1 1 1 1
  spline S291 degree 3 poles (59.7048, 106.6485) (59.6187, 107.5885) (59.4032, 108.5138) (59.3191, 109.4539) knots 0 0 0 0 1 1 1 1
  spline S292 degree 3 poles (59.3191, 109.4539) (59.2911, 109.7664) (59.3068, 110.0863) (59.3697, 110.3936) knots 0 0 0 0 1 1 1 1
  spline S293 degree 3 poles (59.3697, 110.3936) (59.3926, 110.5053) (59.5022, 110.5791) (59.5684, 110.6719) knots 0 0 0 0 1 1 1 1
  spline S294 degree 3 poles (59.5242, 107.6633) (59.6686, 108.1778) (59.8523, 108.6829) (59.9575, 109.2068) knots 0 0 0 0 1 1 1 1
  spline S295 degree 3 poles (59.9575, 109.2068) (60.0046, 109.4415) (59.9155, 109.6936) (59.978, 109.9247) knots 0 0 0 0 1 1 1 1
  spline S296 degree 3 poles (59.978, 109.9247) (60.0004, 110.0077) (60.1077, 110.0484) (60.1908, 110.0702) knots 0 0 0 0 1 1 1 1
  spline S297 degree 3 poles (60.1908, 110.0702) (60.5983, 110.1771) (61.0186, 110.2275) (61.4325, 110.3062) knots 0 0 0 0 1 1 1 1
  spline S298 degree 3 poles (59.3191, 109.4539) (59.2617, 109.053) (59.1807, 108.6547) (59.1469, 108.251) knots 0 0 0 0 1 1 1 1
  spline S299 degree 3 poles (59.1469, 108.251) (59.1217, 107.9512) (59.14, 107.6492) (59.1425, 107.3483) knots 0 0 0 0 1 1 1 1
  spline S300 degree 3 poles (59.1425, 107.3483) (59.2206, 97.9365) (59.2593, 88.5242) (59.3885, 79.1129) knots 0 0 0 0 1 1 1 1
  spline S301 degree 3 poles (59.3885, 79.1129) (59.4, 78.2782) (59.506, 77.4475) (59.5647, 76.6148) knots 0 0 0 0 1 1 1 1
  spline S302 degree 3 poles (59.5029, 101.4584) (59.6109, 101.6641) (59.7189, 101.8699) (59.8268, 102.0757) knots 0 0 0 0 1 1 1 1
  spline S303 degree 3 poles (59.6871, 75.1977) (59.6422, 75.4459) (59.5973, 75.694) (59.5523, 75.9421) knots 0 0 0 0 1 1 1 1
  spline S304 degree 3 poles (59.7076, 79.9703) (59.6333, 78.2715) (59.5333, 76.5735) (59.4847, 74.8737) knots 0 0 0 0 1 1 1 1
  spline S305 degree 3 poles (59.4847, 74.8737) (59.4551, 73.8388) (59.4728, 72.8031) (59.473, 71.7678) knots 0 0 0 0 1 1 1 1
  spline S306 degree 3 poles (59.473, 71.7678) (59.4745, 66.2925) (59.4329, 60.817) (59.4899, 55.342) knots 0 0 0 0 1 1 1 1
  spline S307 degree 3 poles (59.4899, 55.342) (59.5014, 54.247) (59.6155, 53.1555) (59.6782, 52.0623) knots 0 0 0 0 1 1 1 1
  spline S308 degree 3 poles (59.7121, 64.899) (59.7948, 65.3704) (59.9308, 65.8355) (59.9601, 66.3132) knots 0 0 0 0 1 1 1 1
  spline S309 degree 3 poles (59.9601, 66.3132) (60.021, 67.3065) (59.9838, 68.3035) (59.9821, 69.2986) knots 0 0 0 0 1 1 1 1
  spline S310 degree 3 poles (59.9821, 69.2986) (59.9778, 71.7902) (60.0069, 74.2826) (59.9421, 76.7734) knots 0 0 0 0 1 1 1 1
  spline S311 degree 3 poles (59.9421, 76.7734) (59.9161, 77.7728) (59.7873, 78.7668) (59.7099, 79.7635) knots 0 0 0 0 1 1 1 1
  spline S312 degree 3 poles (59.7374, 55.4781) (59.7924, 55.214) (59.8474, 54.9498) (59.9024, 54.6856) knots 0 0 0 0 1 1 1 1
  spline S313 degree 3 poles (59.9601, 66.3132) (59.9336, 65.269) (59.8633, 64.2249) (59.8807, 63.1804) knots 0 0 0 0 1 1 1 1
  spline S314 degree 3 poles (59.8807, 63.1804) (59.8868, 62.8138) (60.0205, 62.4571) (60.0303, 62.0905) knots 0 0 0 0 1 1 1 1
  spline S315 degree 3 poles (60.0303, 62.0905) (60.0885, 59.9112) (60.1222, 57.7302) (60.0846, 55.5505) knots 0 0 0 0 1 1 1 1
  spline S316 degree 3 poles (60.0846, 55.5505) (60.0795, 55.2559) (59.9339, 54.9786) (59.9024, 54.6856) knots 0 0 0 0 1 1 1 1
  spline S317 degree 3 poles (59.9024, 54.6856) (59.7404, 53.1747) (59.5416, 51.6634) (59.5047, 50.1443) knots 0 0 0 0 1 1 1 1
  spline S318 degree 3 poles (59.5047, 50.1443) (59.4954, 49.7625) (59.6782, 49.4005) (59.765, 49.0286) knots 0 0 0 0 1 1 1 1
  spline S319 degree 3 poles (59.7683, 50.2243) (59.7011, 50.523) (59.6339, 50.8218) (59.5667, 51.1205) knots 0 0 0 0 1 1 1 1
  spline S320 degree 3 poles (59.8258, 44.7521) (59.9062, 45.1019) (60.0567, 45.4428) (60.067, 45.8016) knots 0 0 0 0 1 1 1 1
  spline S321 degree 3 poles (60.067, 45.8016) (60.1328, 48.1125) (60.2017, 50.43) (60.0533, 52.737) knots 0 0 0 0 1 1 1 1
  spline S322 degree 3 poles (60.0533, 52.737) (60.0127, 53.368) (59.687, 53.9474) (59.5039, 54.5526) knots 0 0 0 0 1 1 1 1
  spline S323 degree 3 poles (59.7877, 48.5922) (59.7838, 48.3839) (59.804, 48.1737) (59.776, 47.9673) knots 0 0 0 0 1 1 1 1
  spline S324 degree 3 poles (59.776, 47.9673) (59.7363, 47.6752) (59.6489, 47.3917) (59.5854, 47.1039) knots 0 0 0 0 1 1 1 1
  spline S325 degree 3 poles (59.566, 49.735) (59.5553, 49.0321) (59.4973, 48.3283) (59.5339, 47.6262) knots 0 0 0 0 1 1 1 1
  spline S326 degree 3 poles (59.5339, 47.6262) (59.5841, 46.6645) (59.8174, 45.715) (59.8258, 44.7521) knots 0 0 0 0 1 1 1 1
  spline S327 degree 3 poles (59.8258, 44.7521) (59.8453, 42.5018) (59.6228, 40.2545) (59.6175, 38.0041) knots 0 0 0 0 1 1 1 1
  spline S328 degree 3 poles (59.6175, 38.0041) (59.6056, 33.0227) (59.6801, 28.0412) (59.7741, 23.0607) knots 0 0 0 0 1 1 1 1
  spline S329 degree 3 poles (59.7741, 23.0607) (59.7823, 22.6279) (59.8144, 22.1896) (59.9239, 21.7708) knots 0 0 0 0 1 1 1 1
  spline S330 degree 3 poles (59.9239, 21.7708) (59.9897, 21.5189) (60.1931, 21.3228) (60.2912, 21.0816) knots 0 0 0 0 1 1 1 1
  spline S331 degree 3 poles (60.2912, 21.0816) (60.5271, 20.5015) (60.5999, 19.8486) (60.9235, 19.3124) knots 0 0 0 0 1 1 1 1
  spline S332 degree 3 poles (60.9235, 19.3124) (61.0948, 19.0285) (61.454, 18.9144) (61.7193, 18.7154) knots 0 0 0 0 1 1 1 1
  spline S333 degree 3 poles (59.8508, 39.1169) (59.8049, 39.773) (59.759, 40.4292) (59.7131, 41.0853) knots 0 0 0 0 1 1 1 1
  spline S334 degree 3 poles (59.6905, 26.7111) (59.8323, 27.5881) (60.01, 28.46) (60.1159, 29.342) knots 0 0 0 0 1 1 1 1
  spline S335 degree 3 poles (60.1159, 29.342) (60.1598, 29.7078) (60.1401, 30.0787) (60.139, 30.4472) knots 0 0 0 0 1 1 1 1
  spline S336 degree 3 poles (60.139, 30.4472) (60.1263, 34.5128) (60.1689, 38.5794) (60.0744, 42.644) knots 0 0 0 0 1 1 1 1
  spline S337 degree 3 poles (60.0744, 42.644) (60.0659, 43.0099) (59.912, 43.3577) (59.8307, 43.7145) knots 0 0 0 0 1 1 1 1
  spline S338 degree 3 poles (60.2256, 21.9354) (60.2474, 21.6508) (60.2693, 21.3662) (60.2912, 21.0816) knots 0 0 0 0 1 1 1 1
  spline S339 degree 3 poles (60.15, 22.2797) (60.0899, 22.3229) (60.0063, 22.4735) (59.9698, 22.4092) knots 0 0 0 0 1 1 1 1
  spline S340 degree 3 poles (59.9698, 22.4092) (59.8764, 22.2446) (59.9255, 22.0332) (59.9034, 21.8452) knots 0 0 0 0 1 1 1 1
  spline S341 degree 3 poles (62.1405, 16.7113) (62.1136, 16.7812) (62.0406, 16.8487) (62.06, 16.9211) knots 0 0 0 0 1 1 1 1
  spline S342 degree 3 poles (62.06, 16.9211) (62.084, 17.0108) (62.1872, 17.0563) (62.2509, 17.124) knots 0 0 0 0 1 1 1 1
  spline S343 degree 3 poles (61.1594, 18.8061) (62.2643, 15.3684) (63.2584, 11.8931) (64.4741, 8.493) knots 0 0 0 0 1 1 1 1
  spline S344 degree 3 poles (64.4741, 8.493) (64.6264, 8.0672) (64.463, 9.4041) (64.3634, 9.8452) knots 0 0 0 0 1 1 1 1
  spline S345 degree 3 poles (64.3634, 9.8452) (63.957, 11.6449) (63.5258, 13.4432) (62.96, 15.1993) knots 0 0 0 0 1 1 1 1
  spline S346 degree 3 poles (62.96, 15.1993) (62.2355, 17.4475) (61.2561, 19.6069) (60.4972, 21.8437) knots 0 0 0 0 1 1 1 1
  spline S347 degree 3 poles (60.4972, 21.8437) (60.3882, 22.165) (60.3822, 22.5139) (60.3635, 22.8527) knots 0 0 0 0 1 1 1 1
  spline S348 degree 3 poles (60.3635, 22.8527) (60.2901, 24.1818) (60.3583, 25.5196) (60.2211, 26.8437) knots 0 0 0 0 1 1 1 1
  spline S349 degree 3 poles (60.2211, 26.8437) (60.1214, 27.806) (59.8439, 28.7414) (59.6552, 29.6902) knots 0 0 0 0 1 1 1 1
  spline S350 degree 3 poles (68.9026, 65.3628) (68.6451, 65.8616) (68.3877, 66.3604) (68.1302, 66.8592) knots 0 0 0 0 1 1 1 1
  spline S351 degree 3 poles (78.028, 17.5835) (77.9833, 17.2317) (77.9387, 16.8798) (77.894, 16.5279) knots 0 0 0 0 1 1 1 1
  spline S352 degree 3 poles (79.4406, 108.4867) (79.4836, 104.0336) (79.5492, 99.5806) (79.5696, 95.1273) knots 0 0 0 0 1 1 1 1
  spline S353 degree 3 poles (79.5696, 95.1273) (79.5997, 88.5649) (79.5605, 82.0023) (79.5921, 75.4399) knots 0 0 0 0 1 1 1 1
  spline S354 degree 3 poles (79.5921, 75.4399) (79.5986, 74.0791) (79.6123, 72.7174) (79.6839, 71.3585) knots 0 0 0 0 1 1 1 1
  spline S355 degree 3 poles (79.6839, 71.3585) (79.7071, 70.9182) (79.8507, 70.49) (79.8759, 70.0498) knots 0 0 0 0 1 1 1 1
  spline S356 degree 3 poles (79.8759, 70.0498) (79.9167, 69.3391) (79.9234, 68.6249) (79.8815, 67.9143) knots 0 0 0 0 1 1 1 1
  spline S357 degree 3 poles (79.8815, 67.9143) (79.8628, 67.5973) (79.7148, 67.297) (79.6948, 66.98) knots 0 0 0 0 1 1 1 1
  spline S358 degree 3 poles (79.6948, 66.98) (79.6237, 65.8542) (79.5639, 64.7242) (79.6089, 63.597) knots 0 0 0 0 1 1 1 1
  spline S359 degree 3 poles (79.6089, 63.597) (79.6315, 63.033) (79.8008, 62.4844) (79.8967, 61.9281) knots 0 0 0 0 1 1 1 1
  spline S360 degree 3 poles (79.9482, 100.5501) (79.8, 100.5441) (79.6518, 100.538) (79.5037, 100.5319) knots 0 0 0 0 1 1 1 1
  spline S361 degree 3 poles (77.701, 17.4128) (77.783, 17.6687) (77.8339, 17.9367) (77.9469, 18.1806) knots 0 0 0 0 1 1 1 1
  spline S362 degree 3 poles (77.9469, 18.1806) (78.2672, 18.8717) (78.6702, 19.5222) (78.9974, 20.2101) knots 0 0 0 0 1 1 1 1
  spline S363 degree 3 poles (78.9974, 20.2101) (79.1955, 20.6265) (79.3576, 21.0594) (79.5215, 21.4904) knots 0 0 0 0 1 1 1 1
  spline S364 degree 3 poles (79.5215, 21.4904) (79.7375, 22.0587) (79.9702, 22.6226) (80.1367, 23.2073) knots 0 0 0 0 1 1 1 1
  spline S365 degree 3 poles (80.1367, 23.2073) (80.1855, 23.3787) (80.1596, 23.5631) (80.1622, 23.7412) knots 0 0 0 0 1 1 1 1
  spline S366 degree 3 poles (80.1622, 23.7412) (80.1721, 24.4015) (80.2157, 25.0632) (80.1742, 25.7222) knots 0 0 0 0 1 1 1 1
  spline S367 degree 3 poles (80.1742, 25.7222) (80.1461, 26.1686) (79.9725, 26.5991) (79.9543, 27.046) knots 0 0 0 0 1 1 1 1
  spline S368 degree 3 poles (79.9543, 27.046) (79.8157, 30.4449) (79.7716, 33.8469) (79.7042, 37.2479) knots 0 0 0 0 1 1 1 1
  spline S369 degree 3 poles (79.7042, 37.2479) (79.6948, 37.7201) (79.6934, 38.1933) (79.724, 38.6645) knots 0 0 0 0 1 1 1 1
  spline S370 degree 3 poles (79.724, 38.6645) (79.7347, 38.8289) (79.8273, 38.983) (79.8275, 39.1477) knots 0 0 0 0 1 1 1 1
  spline S371 degree 3 poles (79.8275, 39.1477) (79.8278, 39.3911) (79.7296, 39.6275) (79.7256, 39.8709) knots 0 0 0 0 1 1 1 1
  spline S372 degree 3 poles (79.7256, 39.8709) (79.6923, 41.9332) (79.6571, 43.9967) (79.7159, 46.0584) knots 0 0 0 0 1 1 1 1
  spline S373 degree 3 poles (79.7159, 46.0584) (79.7261, 46.4178) (79.8961, 46.7574) (79.9323, 47.1152) knots 0 0 0 0 1 1 1 1
  spline S374 degree 3 poles (79.9323, 47.1152) (79.9678, 47.4654) (79.9616, 47.8208) (79.9298, 48.1714) knots 0 0 0 0 1 1 1 1
  spline S375 degree 3 poles (79.9298, 48.1714) (79.8867, 48.6449) (79.7388, 49.106) (79.7082, 49.5804) knots 0 0 0 0 1 1 1 1
  spline S376 degree 3 poles (79.7082, 49.5804) (79.6579, 50.3602) (79.6867, 51.1431) (79.6877, 51.9245) knots 0 0 0 0 1 1 1 1
  spline S377 degree 3 poles (79.6877, 51.9245) (79.6888, 52.7859) (79.6652, 53.6486) (79.7144, 54.5086) knots 0 0 0 0 1 1 1 1
  spline S378 degree 3 poles (79.7144, 54.5086) (79.7399, 54.9549) (79.9004, 55.3883) (79.9114, 55.8352) knots 0 0 0 0 1 1 1 1
  spline S379 degree 3 poles (79.9114, 55.8352) (79.9613, 57.8656) (79.8428, 59.8979) (79.8967, 61.9281) knots 0 0 0 0 1 1 1 1
  spline S380 degree 3 poles (79.8967, 61.9281) (79.9132, 62.5498) (80.0742, 63.16) (80.1224, 63.7799) knots 0 0 0 0 1 1 1 1
  spline S381 degree 3 poles (80.1224, 63.7799) (80.1421, 64.0321) (80.1481, 64.29) (80.0998, 64.5383) knots 0 0 0 0 1 1 1 1
  spline S382 degree 3 poles (80.0998, 64.5383) (80.005, 65.0261) (79.8307, 65.4951) (79.6961, 65.9736) knots 0 0 0 0 1 1 1 1
  spline S383 degree 3 poles (79.9977, 41.3411) (80.0603, 40.6933) (80.1229, 40.0455) (80.1855, 39.3976) knots 0 0 0 0 1 1 1 1
  spline S384 degree 3 poles (79.9551, 30.2867) (79.9567, 29.9023) (79.8155, 29.4897) (79.9599, 29.1335) knots 0 0 0 0 1 1 1 1
  spline S385 degree 3 poles (79.9599, 29.1335) (80.0407, 28.9342) (80.1728, 29.5262) (80.1763, 29.7412) knots 0 0 0 0 1 1 1 1
  spline S386 degree 3 poles (80.1763, 29.7412) (80.2572, 34.7303) (80.2084, 39.7207) (80.2123, 44.7105) knots 0 0 0 0 1 1 1 1
  spline S387 degree 3 poles (80.2123, 44.7105) (80.2127, 45.1483) (80.2399, 45.5889) (80.1892, 46.0238) knots 0 0 0 0 1 1 1 1
  spline S388 degree 3 poles (80.1892, 46.0238) (80.146, 46.395) (80.0179, 46.7514) (79.9323, 47.1152) knots 0 0 0 0 1 1 1 1
  spline S389 degree 3 poles (79.8627, 25.8921) (79.816, 25.5724) (79.7307, 25.256) (79.7226, 24.933) knots 0 0 0 0 1 1 1 1
  spline S390 degree 3 poles (79.7226, 24.933) (79.7004, 24.0516) (79.7555, 23.1699) (79.7719, 22.2884) knots 0 0 0 0 1 1 1 1
  spline S391 degree 3 poles (77.1865, 15.9589) (77.2957, 16.2902) (77.3341, 16.654) (77.514, 16.9528) knots 0 0 0 0 1 1 1 1
  spline S392 degree 3 poles (77.514, 16.9528) (77.7854, 17.4038) (78.1834, 17.7653) (78.5181, 18.1715) knots 0 0 0 0 1 1 1 1
  spline S393 degree 3 poles (77.894, 16.5279) (77.6267, 16.2248) (77.2672, 15.9827) (77.092, 15.6185) knots 0 0 0 0 1 1 1 1